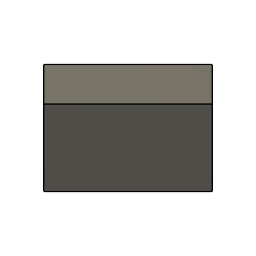
box_ry45_run01 (Autodesk Fusion 360 design; units mm, degrees)
Autodesk Fusion 360 part; units mm, degrees
ref_plane "工作平面1" through (0, 12.125, 0) normal (0.707107, 0, 0.707107) x (0, 1, 0)
sketch "草图1" plane through (0, 0, 0) normal (0.707107, 0, 0.707107) x (0, 1, 0)
  line L0 (0, 0) -> (0, -44)
  line L1 (0, -44) -> (28, -44)
  line L2 (28, -44) -> (28, 0)
  line L3 (28, 0) -> (0, 0)
extrude "拉伸1" add sketch "草图1" along normal blind 18
